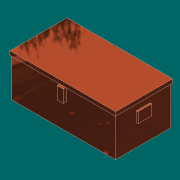
# Autodesk Inventor part: Jobox tool box
Saved by Autodesk Inventor 2017 (Build 210142000, 142)
## iProperties
Created: 2018-01-23
Part Number: Jobox tool box
Material: Copper
Document SubType Name: Modeling
Designer: Graeme_Van_Dongen
Density: 8.94 g/cm^3
Appearance: Copper - Satin
Author: Graeme_Van_Dongen
Autodesk Inventor part; units mm, degrees
ref_plane "YZ Plane" through (0, 0, 0) normal (1, 0, 0) x (0, 1, 0)
ref_plane "XZ Plane" through (0, 0, 0) normal (0, 1, 0) x (-1, 0, 0)
ref_plane "XY Plane" through (0, 0, 0) normal (0, 0, 1) x (1, 0, 0)
sketch "Sketch1" plane through (0, 0, 0) normal (0, 1, 0) x (-1, 0, 0)
  line L0 (381, 203.2) -> (-381, 203.2)
  line L1 (-381, 203.2) -> (-381, -203.2)
  line L2 (-381, -203.2) -> (381, -203.2)
  line L3 (381, -203.2) -> (381, 203.2)
  line L4 (381, 203.2) -> (-381, -203.2) construction
  line L5 (-381, 203.2) -> (381, -203.2) construction
  point P0 (0, 0)
  dimension "d0" = 762
  dimension "d1" = 406.4
  constraints: 12 end point, 2 midpoint, 2 parallel, 1 horizontal, 1 perpendicular
  measures "d0" distance of L2.end L1.end
  measures "d1" distance of L1.end L0.end
extrude "Extrusion1" add sketch "Sketch1" along normal blind 311.15
sketch "Sketch2" plane through (0, 311.15, 0) normal (0, 1, 0) x (1, 0, 0)
  line L0 (-387.35, -209.55) -> (387.35, -209.55)
  line L1 (387.35, -209.55) -> (387.35, 209.55)
  line L2 (387.35, 209.55) -> (-387.35, 209.55)
  line L3 (-387.35, 209.55) -> (-387.35, -209.55)
  line L4 (-387.35, -209.55) -> (387.35, 209.55) construction
  line L5 (387.35, -209.55) -> (-387.35, 209.55) construction
  point P0 (-381, -203.2)
  point P1 (381, -203.2)
  point P2 (0, 0)
  dimension "d20" = 774.7
  dimension "d21" = 419.1
  constraints: 12 end point, 2 midpoint, 2 parallel, 1 horizontal, 1 perpendicular
  measures "d20" distance of L2.end L1.end
  measures "d21" distance of L1.end L0.end
extrude "Extrusion2" add sketch "Sketch2" against normal blind 28.575
sketch "Sketch3" plane through (-381, 0, 203.2) normal (0, 0, 1) x (1, 0, 0)
  line L0 (358.775, 190.5) -> (403.225, 190.5)
  line L1 (403.225, 190.5) -> (403.225, 282.575)
  line L2 (403.225, 282.575) -> (358.775, 282.575)
  line L3 (358.775, 282.575) -> (358.775, 190.5)
  line L4 (762, 282.575) -> (0, 282.575) construction
  point P0 (381, 0)
  point P1 (381, 190.5)
  dimension "d7" = 44.45
  dimension "d8" = 190.5
  constraints: 8 end point, 2 parallel, 1 collinear, 1 horizontal, 1 midpoint, 1 perpendicular, 1 vertical alignment
  measures "d7" distance of L2.end L1.end
  measures "d8" distance from line of L0 point (381, 0)
extrude "Extrusion3" add sketch "Sketch3" along normal blind 25.4
sketch "Sketch4" plane through (381, 0, 203.2) normal (1, 0, 0) x (0, 0, -1)
  line L0 (152.4, 158.75) -> (254, 158.75)
  line L1 (254, 158.75) -> (254, 234.95)
  line L2 (254, 234.95) -> (152.4, 234.95)
  line L3 (152.4, 234.95) -> (152.4, 158.75)
  point P0 (203.2, 0)
  point P1 (203.2, 158.75)
  dimension "d11" = 101.6
  dimension "d12" = 158.75
  dimension "d13" = 76.2
  constraints: 8 end point, 2 parallel, 1 horizontal, 1 midpoint, 1 perpendicular, 1 vertical alignment
  measures "d11" distance of L2.end L1.end
  measures "d12" distance from line of point (203.2, 0) L0
  measures "d13" distance of L0.end L1.end
extrude "Extrusion4" add sketch "Sketch4" along normal blind 12.7
mirror "Mirror1" about plane through (0, 0, 0) normal (1, 0, 0) of "Extrusion4"
body "Solid1"
